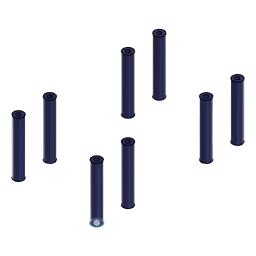
Support poles (Autodesk Fusion 360 design; units mm, degrees)
Autodesk Fusion 360 part; units mm, degrees
sketch "sketch 536" plane through (0, 0, 8) normal (0, 0, 1) x (-1, 0, 0)
  circle A0 centre (-230, 90) radius 2.5
  circle A1 centre (-230, 90) radius 6
extrude "Extrude1" add sketch "sketch 536" along normal blind 70 makes body 1
copy_body "CopyPasteBodies1" bodies 1 makes body 2
move_body "Move1" bodies 2 to x (1, 0, 0) y (0, 1, 0) z (0, 0, 1) at (0, 40, 0)
copy_body "CopyPasteBodies2" bodies 2 1 makes body 3 makes body 4
move_body "Move2" bodies 3 4 to x (1, 0, 0) y (0, 1, 0) z (0, 0, 1) at (-100, 0, 0)
copy_body "CopyPasteBodies3" bodies 4 3 1 2 makes body 5 makes body 6 makes body 7 makes body 8
move_body "Move3" bodies 5 6 7 8 to x (1, 0, 0) y (0, 1, 0) z (0, 0, 1) at (0, 140, 0)
